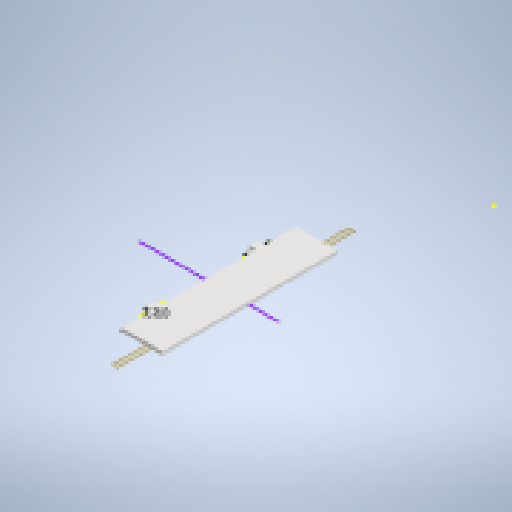
# Autodesk Inventor part: крепление Y
Saved by Autodesk Inventor 2024.2 (Build 282272000, 272)
## iProperties
Created: 2026-02-01
Part Number: крепление Y
Material: Типовые
Document SubType Name: Modeling
Designer: katya_notebook
Density: 1 g/cm^3
Appearance: По умолчанию
Author: katya_notebook
Autodesk Inventor part; units mm, degrees
ref_plane "YZ Plane" through (0, 0, 0) normal (1, 0, 0) x (0, 1, 0)
ref_plane "XZ Plane" through (0, 0, 0) normal (0, 1, 0) x (-1, 0, 0)
ref_plane "XY Plane" through (0, 0, 0) normal (0, 0, 1) x (1, 0, 0)
ref_plane "РабПлоскость1" through (-53.4845, 288.2505, 354.5129) normal (0, 1, 0) x (-1, 0, 0)
sketch "Эскиз1" plane through (-53.4845, 288.2505, 354.5129) normal (0, 1, 0) x (-1, 0, 0)
  line L0 (32.7, -62.75) -> (32.7, -56.5) projected
  line L1 (-13.3, 0) -> (-13.3, -240) projected
  line L2 (-13.3, -220) -> (32.7, -220)
  line L3 (32.7, -220) -> (32.7, -25)
  line L4 (32.7, -25) -> (-13.3, -25)
  line L5 (-13.3, -25) -> (-13.3, -220)
  line L6 (-5.3, -220) -> (142.8907, -220) projected
  line L7 (201.7, -25) -> (-5.3, -25) projected
  point P0 (-53.4845, -354.5129)
  point P1 (-13.3, -25)
  point P2 (-13.3, -220)
  constraints: 8 end point, 2 parallel, 2 point on line, 1 horizontal, 1 perpendicular
extrude "Выдавливание1" add sketch "Эскиз1" along normal blind 4
sketch "Эскиз2" plane through (-53.4845, 288.2505, 354.5129) normal (0, -1, 0) x (1, 0, 0)
  line L0 (-32.7, -165.5) -> (-32.7, -172.5) projected
  line L1 (-32.7, -165.5) -> (-38.7, -165.5) projected
  line L2 (-38.7, -172.5) -> (-38.7, -165.5) projected
  line L3 (-32.7, -172.5) -> (-38.7, -172.5) projected
  line L4 (-32.7, -188.5) -> (-32.7, -195.5) projected
  line L5 (-32.7, -188.5) -> (-38.7, -188.5) projected
  line L6 (-38.7, -195.5) -> (-38.7, -188.5) projected
  line L7 (-32.7, -195.5) -> (-38.7, -195.5) projected
  circle A0 centre (-35.7, -180.5) radius 1.75 projected
  line L8 (-37.8999, -64.576) -> (-32.1499, -64.576) projected
  circle A1 centre (-35.7, -64.5) radius 1.75 projected
  line L9 (-38.7, -79.5) -> (-38.7, -72.5) projected
  line L10 (-32.7, -72.5) -> (-32.7, -79.5) projected
  line L11 (-38.7, -56.5) -> (-38.7, -49.5) projected
  line L12 (-32.8499, -56.124) -> (-32.8499, -45.124) projected
  line L13 (-32.7, -49.5) -> (-38.7, -49.5) projected
  line L14 (-32.7, -220) -> (-32.7, -25) projected
  line L15 (-32.7, -59.324) -> (-30.2517, -59.324)
  line L16 (-30.2517, -59.324) -> (-30.2517, -69.324)
  line L17 (-30.2517, -69.324) -> (-32.7, -69.324)
  line L18 (-32.7, -69.324) -> (-32.7, -59.324)
  line L19 (-111.002, -122.5) -> (45.2006, -122.5)
  line L20 (-37.8999, -180.424) -> (-32.1499, -180.424)
  circle A2 centre (-35.7, -180.5) radius 1.75
  line L21 (-38.7, -165.5) -> (-38.7, -172.5)
  line L22 (-32.7, -172.5) -> (-32.7, -165.5)
  line L23 (-38.7, -188.5) -> (-38.7, -195.5)
  line L24 (-32.8499, -188.876) -> (-32.8499, -199.876)
  line L25 (-32.7, -195.5) -> (-38.7, -195.5)
  line L26 (-32.7, -25) -> (-32.7, -220)
  line L27 (-32.7, -185.676) -> (-30.2517, -185.676)
  line L28 (-30.2517, -185.676) -> (-30.2517, -175.676)
  line L29 (-30.2517, -175.676) -> (-32.7, -175.676)
  line L30 (-32.7, -175.676) -> (-32.7, -185.676)
  point P0 (53.4845, -354.5129)
  dimension "d2" = 10
  dimension "d3" = 3.2
  constraints: 32 end point, 11 symmetric about line, 2 horizontal, 2 parallel, 1 centre point, 1 perpendicular, 1 point on line, 4 other
  measures "d2" distance of L15.end L16.end
  measures "d3" vertical distance of L15.start L12.start
sketch "Эскиз3" plane through (-86.1845, 288.2505, 134.5129) normal (-1, 0, 0) x (0, 0, 1)
  line L0 (0, 0) -> (195, 0) projected
  line L1 (0, 4) -> (195, 4) projected
  line L2 (44.3461, 0) -> (34.3461, 0)
  line L3 (34.3461, 0) -> (34.3461, 4)
  line L4 (34.3461, 4) -> (44.3461, 4)
  line L5 (44.3461, 4) -> (44.3461, 0)
  line L6 (160.6836, 0) -> (150.6836, 0)
  line L7 (150.6836, 0) -> (150.6836, 4)
  line L8 (150.6836, 4) -> (160.6836, 4)
  line L9 (160.6836, 4) -> (160.6836, 0)
  point P0 (-134.5129, -288.2505)
  point P1 (44.3461, 4)
  point P2 (34.3461, 0)
  point P3 (160.6836, 4)
  point P4 (150.6836, 0)
  dimension "d4" = 10
  dimension "d5" = 10
  constraints: 16 end point, 4 parallel, 4 point on line, 2 horizontal, 2 perpendicular
  measures "d4" distance of L3.end L4.end
  measures "d5" distance of L7.end L8.end
extrude "Выдавливание2" add sketch "Эскиз3" along normal blind 8 contours L3 L1 L5 L0 | L7 L1 L9 L0
sketch "Эскиз4" plane through (-53.4845, 288.2505, 354.5129) normal (0, -1, 0) x (1, 0, 0)
  point P0 (53.4845, -354.5129)
